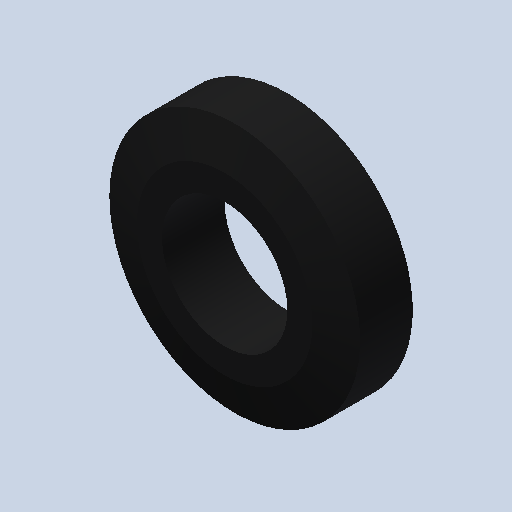
# Autodesk Inventor part: SPACER,BEARING,SLIDE,TOP,ELEVATOR
Saved by Autodesk Inventor 2025.2 (Build 292293000, 293)
## iProperties
Category: _
Manager: _
ILogicPurgeVersion: 0.0.0.0
OnSaveVersion: 3.4.3.0
OnSaveAssembly: COREAutomationManager
Created: 2025-01-27
Part Number: SPACER,BEARING,SLIDE,TOP,ELEVATOR
Checked By: 00
Engr Approved By: _
User Status: Work In Process
Material: 3D Print Material - chopped carbon Nylon12 (preferred)
Description: STANDARD (mm)
Document SubType Name: Modeling
Mfg Approved By: John.Thibert
Designer: John.Thibert
Manufacturer: Standard
Standards Organization: Custom
Density: 1.05184 g/cm^3
Appearance: Black
CN_MASS: 0.0
CN_SERVICEABLE: _
FIRST_DESCRIPTION: _
SECOND_DESCRIPTION: _
THIRD_DESCRIPTION: _
ModelCat: Uncategorized
MaterialName: 3D Print Material - chopped carbon Nylon12 (preferred)
Subject: _
Author: John.Thibert
Keywords: -
Revision Number: A
Autodesk Inventor part; units mm, degrees
ref_plane "YZ Plane" through (0, 0, 0) normal (1, 0, 0) x (0, 1, 0)
ref_plane "XZ Plane" through (0, 0, 0) normal (0, 1, 0) x (-1, 0, 0)
ref_plane "XY Plane" through (0, 0, 0) normal (0, 0, 1) x (1, 0, 0)
sketch "Sketch2" plane through (0, 0, 0) normal (0, 1, 0) x (-1, 0, 0)
  line L0 (3.175, -1.5875) -> (3.175, 1.5875)
  line L1 (6.35, 1.0771) -> (6.35, -1.5875)
  line L2 (6.35, -1.5875) -> (3.175, -1.5875)
  line L3 (0, -2.2225) -> (0, 2.2225) construction
  line L4 (3.175, 1.5875) -> (4.445, 1.5875)
  line L5 (4.445, 1.5875) -> (6.35, 1.0771)
  point P0 (0, 0)
  point P1 (3.175, 0)
  dimension "d0" = 6.35
  dimension "d1" = 12.7
  dimension "d7" = 3.175
  dimension "d8" = 15
  dimension "d9" = 1.27
  constraints: 10 end point, 1 horizontal, 1 horizontal alignment, 1 midpoint, 1 perpendicular, 1 vertical
  measures "d0" diameter of L0 L3
  measures "d1" diameter of L1 L3
  measures "d7" distance of L0.start L0.end
  measures "d8" angle of L4 L5
  measures "d9" distance of L0.end L4.end
revolve "Revolution1" add sketch "Sketch2" angle 360 about axis through (0, 0, -10) along (0, 0, 1)
body "Solid1"
